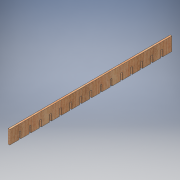
# Autodesk Inventor part: DividerWidth
Saved by Autodesk Inventor 2016 (Build 200138000, 138)
## iProperties
Created: 2016-02-08
Part Number: DividerWidth
Material: Wood (Birch)
Document SubType Name: Modeling
Designer: ron
Density: 0.55 g/cm^3
Appearance: Birch - Natural Polished
Mass: 99.705 g
Surface Area: 703.224 cm^2
Volume: 181.282 cm^3
Author: ron
Autodesk Inventor part; units mm, degrees
ref_plane "YZ Plane" through (0, 0, 0) normal (1, 0, 0) x (0, 1, 0)
ref_plane "XZ Plane" through (0, 0, 0) normal (0, 1, 0) x (-1, 0, 0)
ref_plane "XY Plane" through (0, 0, 0) normal (0, 0, 1) x (1, 0, 0)
sketch "Sketch1" plane through (0, 0, 0) normal (1, 0, 0) x (0, 1, 0)
  line L0 (0, 0) -> (50.8, 0)
  line L1 (50.8, 0) -> (50.8, -609.6)
  line L2 (50.8, -609.6) -> (0, -609.6)
  line L3 (0, -609.6) -> (0, -574.675)
  line L4 (0, -574.675) -> (25.4, -574.675)
  line L5 (25.4, -574.675) -> (25.4, -568.325)
  line L6 (25.4, -568.325) -> (0, -568.325)
  line L7 (0, -568.325) -> (0, -536.575)
  line L8 (0, -536.575) -> (25.4, -536.575)
  line L9 (25.4, -536.575) -> (25.4, -530.225)
  line L10 (25.4, -530.225) -> (0, -530.225)
  line L11 (0, -530.225) -> (0, -498.475)
  line L12 (0, -498.475) -> (25.4, -498.475)
  line L13 (25.4, -498.475) -> (25.4, -492.125)
  line L14 (25.4, -492.125) -> (0, -492.125)
  line L15 (0, -492.125) -> (0, -460.375)
  line L16 (0, -460.375) -> (25.4, -460.375)
  line L17 (25.4, -460.375) -> (25.4, -454.025)
  line L18 (25.4, -454.025) -> (0, -454.025)
  line L19 (0, -454.025) -> (0, -422.275)
  line L20 (0, -422.275) -> (25.4, -422.275)
  line L21 (25.4, -422.275) -> (25.4, -415.925)
  line L22 (25.4, -415.925) -> (0, -415.925)
  line L23 (0, -415.925) -> (0, -384.175)
  line L24 (0, -384.175) -> (25.4, -384.175)
  line L25 (25.4, -384.175) -> (25.4, -377.825)
  line L26 (25.4, -377.825) -> (0, -377.825)
  line L27 (0, -377.825) -> (0, -346.075)
  line L28 (0, -346.075) -> (25.4, -346.075)
  line L29 (25.4, -346.075) -> (25.4, -339.725)
  line L30 (25.4, -339.725) -> (0, -339.725)
  line L31 (0, -339.725) -> (0, -307.975)
  line L32 (0, -307.975) -> (25.4, -307.975)
  line L33 (25.4, -307.975) -> (25.4, -301.625)
  line L34 (25.4, -301.625) -> (0, -301.625)
  line L35 (0, -301.625) -> (0, -269.875)
  line L36 (0, -269.875) -> (25.4, -269.875)
  line L37 (25.4, -269.875) -> (25.4, -263.525)
  line L38 (25.4, -263.525) -> (0, -263.525)
  line L39 (0, -263.525) -> (0, -231.775)
  line L40 (0, -231.775) -> (25.4, -231.775)
  line L41 (25.4, -231.775) -> (25.4, -225.425)
  line L42 (25.4, -225.425) -> (0, -225.425)
  line L43 (0, -225.425) -> (0, -193.675)
  line L44 (0, -193.675) -> (25.4, -193.675)
  line L45 (25.4, -193.675) -> (25.4, -187.325)
  line L46 (25.4, -187.325) -> (0, -187.325)
  line L47 (0, -187.325) -> (0, -155.575)
  line L48 (0, -155.575) -> (25.4, -155.575)
  line L49 (25.4, -155.575) -> (25.4, -149.225)
  line L50 (25.4, -149.225) -> (0, -149.225)
  line L51 (0, -149.225) -> (0, -117.475)
  line L52 (0, -117.475) -> (25.4, -117.475)
  line L53 (25.4, -117.475) -> (25.4, -111.125)
  line L54 (25.4, -111.125) -> (0, -111.125)
  line L55 (0, -111.125) -> (0, -79.375)
  line L56 (0, -79.375) -> (25.4, -79.375)
  line L57 (25.4, -79.375) -> (25.4, -73.025)
  line L58 (25.4, -73.025) -> (0, -73.025)
  line L59 (0, -73.025) -> (0, -41.275)
  line L60 (0, -41.275) -> (25.4, -41.275)
  line L61 (25.4, -41.275) -> (25.4, -34.925)
  line L62 (25.4, -34.925) -> (0, -34.925)
  line L63 (0, 0) -> (0, -34.925)
  dimension "d293" = 50.8
  dimension "d294" = 609.6
  dimension "d295" = 34.925
  dimension "d296" = 25.4
  dimension "d297" = 6.35
  dimension "d298" = 25.4
  dimension "d299" = 31.75
  dimension "d300" = 6.35
  dimension "d301" = 31.75
  dimension "d302" = 6.35
  dimension "d303" = 31.75
  dimension "d304" = 6.35
  dimension "d305" = 31.75
  dimension "d306" = 6.35
  dimension "d307" = 31.75
  dimension "d308" = 6.35
  dimension "d309" = 31.75
  dimension "d310" = 6.35
  dimension "d311" = 31.75
  dimension "d312" = 6.35
  dimension "d313" = 31.75
  dimension "d314" = 6.35
  dimension "d315" = 31.75
  dimension "d316" = 6.35
  dimension "d317" = 31.75
  dimension "d318" = 6.35
  dimension "d319" = 31.75
  dimension "d320" = 6.35
  dimension "d321" = 31.75
  dimension "d322" = 6.35
  dimension "d323" = 31.75
  dimension "d324" = 6.35
  dimension "d325" = 31.75
  dimension "d326" = 6.35
  dimension "d327" = 34.925
  dimension "d328" = 90
  dimension "d329" = 90
  dimension "d330" = 90
  dimension "d331" = 90
  dimension "d332" = 90
  dimension "d333" = 90
  dimension "d334" = 90
  dimension "d335" = 90
  dimension "d336" = 90
  dimension "d337" = 90
  dimension "d338" = 90
  dimension "d339" = 25.4
  dimension "d340" = 25.4
  dimension "d341" = 50.8
  dimension "d342" = 50.8
  dimension "d343" = 50.8
  dimension "d344" = 50.8
  dimension "d345" = 50.8
  dimension "d346" = 50.8
  dimension "d347" = 50.8
  dimension "d348" = 50.8
  dimension "d349" = 50.8
  dimension "d350" = 50.8
  dimension "d351" = 50.8
  dimension "d352" = 50.8
  dimension "d353" = 50.8
  dimension "d354" = 25.4
  dimension "d355" = 25.4
  dimension "d356" = 25.4
  constraints: 128 end point, 19 perpendicular, 15 horizontal, 14 parallel, 4 point on line, 1 vertical
  measures "d293" distance of L0.start L0.end
  measures "d294" distance of L0.end L1.end
  measures "d295" distance of L2.end L3.end
  measures "d296" distance of L3.end L4.end
  measures "d297" distance of L4.end L5.end
  measures "d298" distance of L5.end L6.end
  measures "d299" distance of L6.end L7.end
  measures "d300" distance of L8.end L9.end
  measures "d301" distance of L10.end L12.start
  measures "d302" distance of L12.end L13.end
  measures "d303" distance of L14.end L16.start
  measures "d304" distance of L16.end L17.end
  measures "d305" distance of L18.end L20.start
  measures "d306" distance of L20.end L21.end
  measures "d307" distance of L22.end L24.start
  measures "d308" distance of L24.end L25.end
  measures "d309" distance of L26.end L28.start
  measures "d310" distance of L28.end L29.end
  measures "d311" distance of L30.end L32.start
  measures "d312" distance of L32.end L33.end
  measures "d313" distance of L34.end L36.start
  measures "d314" distance of L36.end L37.end
  measures "d315" distance of L38.end L40.start
  measures "d316" distance of L40.end L41.end
  measures "d317" distance of L42.end L44.start
  measures "d318" distance of L44.end L45.end
  measures "d319" distance of L46.end L48.start
  measures "d320" distance of L48.end L49.end
  measures "d321" distance of L50.end L52.start
  measures "d322" distance of L52.end L53.end
  measures "d323" distance of L54.end L56.start
  measures "d324" distance of L56.end L57.end
  measures "d325" distance of L58.end L60.start
  measures "d326" distance of L60.end L61.end
  measures "d327" distance of L0.start L62.end
  measures "d328" angle of L61 L0
  measures "d329" angle of L53 L0
  measures "d330" angle of L49 L0
  measures "d331" angle of L45 L0
  measures "d332" angle of L41 L0
  measures "d333" angle of L37 L0
  measures "d334" angle of L33 L0
  measures "d335" angle of L29 L0
  measures "d336" angle of L25 L0
  measures "d337" angle of L21 L0
  measures "d338" angle of L17 L0
  measures "d339" distance between parallel lines of L57 L1
  measures "d340" distance between parallel lines of L5 L1
  measures "d341" distance between parallel lines of L59 L1
  measures "d342" distance between parallel lines of L55 L1
  measures "d343" distance between parallel lines of L51 L1
  measures "d344" distance between parallel lines of L47 L1
  measures "d345" distance between parallel lines of L43 L1
  measures "d346" distance between parallel lines of L39 L1
  measures "d347" distance between parallel lines of L35 L1
  measures "d348" distance between parallel lines of L31 L1
  measures "d349" distance between parallel lines of L27 L1
  measures "d350" distance between parallel lines of L23 L1
  measures "d351" distance between parallel lines of L19 L1
  measures "d352" distance between parallel lines of L15 L1
  measures "d353" distance between parallel lines of L11 L1
  measures "d354" distance from line of L0.start L61
  measures "d355" distance from line of L0.start L53
  measures "d356" distance from line of L0.start L49
extrude "Extrusion2" add sketch "Sketch1" along normal blind 6.35
body "Solid2"
